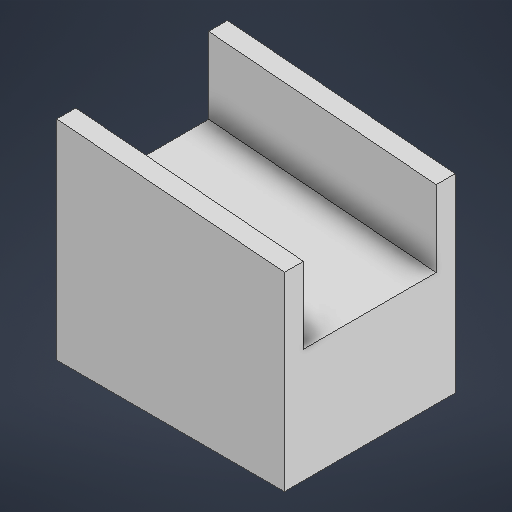
# Autodesk Inventor part: collectionslideintoscrew
Saved by Autodesk Inventor 2026.2 (Build 302298000, 298)
## iProperties
Created: 2026-04-16
Part Number: collectionslideintoscrew
Material: Generic
Document SubType Name: Modeling
Designer: danda
Density: 1 g/cm^3
Appearance: Default
Author: danda
Autodesk Inventor part; units mm, degrees
ref_plane "YZ Plane" through (0, 0, 0) normal (1, 0, 0) x (0, 1, 0)
ref_plane "XZ Plane" through (0, 0, 0) normal (0, 1, 0) x (-1, 0, 0)
ref_plane "XY Plane" through (0, 0, 0) normal (0, 0, 1) x (1, 0, 0)
sketch "Sketch1" plane through (0, 0, 0) normal (0, 0, 1) x (1, 0, 0)
  line L0 (9.2486, 13.3739) -> (9.2486, 48.3739)
  line L1 (9.2486, 13.3739) -> (69.2486, 13.3739)
  line L2 (69.2486, 13.3739) -> (69.2486, 43.3739)
  line L3 (69.2486, 43.3739) -> (9.2486, 48.3739)
  line L4 (69.2486, 63.4432) -> (9.2486, 68.4432)
  line L5 (9.2486, 48.3739) -> (9.2486, 68.4432)
  line L6 (69.2486, 43.3739) -> (69.2486, 63.4432)
  point P0 (0, 0)
  dimension "d0" = 35
  dimension "d1" = 60
  dimension "d2" = 30
  dimension "d3" = 20
  constraints: 14 end point, 3 vertical, 1 horizontal, 1 perpendicular
  measures "d0" distance of L0.start L0.end
  measures "d1" distance of L0.start L1.end
  measures "d2" distance of L1.end L2.end
  measures "d3" distance between parallel lines of L3 L4
extrude "Extrusion1" add sketch "Sketch1" along normal blind 40 and the other way blind 5 contours L0 L3 L2 L1
extrude "Extrusion2" add sketch "Sketch1" against normal blind 5 contours L5 L4 L6 L3
extrude "Extrusion3" add sketch "Sketch1" along normal blind 40 contours L5 L4 L6 L3
extrude "Extrusion4" cut sketch "Sketch1" along normal blind 35 contours L5 L4 L6 L3
body "Solid1"
